Autodesk Inventor part; units mm, degrees
(part 3 of 3)
  spline S534 degree 2 poles (14.1065, -35.038) (14.0102, -34.9886) (13.7829, -34.959) (13.573, -34.959) knots 0 0 0 1 2 2 2
  line L552 (13.573, -34.959) -> (13.1135, -34.959)
  line L553 (13.1135, -34.959) -> (13.1135, -36.0853)
  line L554 (13.1135, -36.0853) -> (13.4421, -36.0853)
  spline S535 degree 2 poles (13.4421, -36.0853) (13.7088, -36.0853) (14.0151, -36.0359) (14.1337, -35.9568) knots 0 0 0 1 2 2 2
  spline S536 degree 2 poles (14.1337, -35.9568) (14.2473, -35.8753) (14.3535, -35.6728) (14.3535, -35.5122) knots 0 0 0 1 2 2 2
  spline S537 degree 2 poles (14.2102, -34.1266) (14.2102, -34.0179) (14.1361, -33.8549) (14.0546, -33.8079) knots 0 0 0 1 2 2 2
  spline S538 degree 2 poles (14.0546, -33.8079) (13.9558, -33.7536) (13.7162, -33.7289) (13.5013, -33.7289) knots 0 0 0 1 2 2 2
  line L555 (13.5013, -33.7289) -> (13.1135, -33.7289)
  line L556 (13.1135, -33.7289) -> (13.1135, -34.6206)
  line L557 (13.1135, -34.6206) -> (13.573, -34.6206)
  spline S539 degree 2 poles (13.573, -34.6206) (13.7632, -34.6206) (13.9435, -34.581) (14.0398, -34.5193) knots 0 0 0 1 2 2 2
  spline S540 degree 2 poles (14.0398, -34.5193) (14.1337, -34.46) (14.2102, -34.2698) (14.2102, -34.1266) knots 0 0 0 1 2 2 2
  spline S541 degree 2 poles (16.4234, -36.189) (16.3764, -36.2236) (16.2184, -36.3471) (16.1443, -36.3841) knots 0 0 0 1 2 2 2
  spline S542 degree 2 poles (16.1443, -36.3841) (16.043, -36.4385) (15.8528, -36.4953) (15.6799, -36.4953) knots 0 0 0 1 2 2 2
  spline S543 degree 2 poles (15.6799, -36.4953) (15.5391, -36.4953) (15.2847, -36.3891) (15.1884, -36.2928) knots 0 0 0 1 2 2 2
  spline S544 degree 2 poles (15.1884, -36.2928) (15.097, -36.1989) (14.9858, -35.9223) (14.9858, -35.7691) knots 0 0 0 1 2 2 2
  spline S545 degree 2 poles (14.9858, -35.7691) (14.9858, -35.532) (15.1859, -35.1961) (15.4032, -35.0997) knots 0 0 0 1 2 2 2
  spline S546 degree 2 poles (15.4032, -35.0997) (15.5959, -35.0108) (16.1195, -34.9441) (16.4234, -34.9268) knots 0 0 0 1 2 2 2
  line L558 (16.4234, -34.9268) -> (16.4234, -34.8527)
  spline S547 degree 2 poles (16.4234, -34.8527) (16.4234, -34.7194) (16.3419, -34.5539) (16.2678, -34.5069) knots 0 0 0 1 2 2 2
  spline S548 degree 2 poles (16.2678, -34.5069) (16.1937, -34.46) (15.9812, -34.4304) (15.8676, -34.4304) knots 0 0 0 1 2 2 2
  spline S549 degree 2 poles (15.8676, -34.4304) (15.7342, -34.4304) (15.3736, -34.5094) (15.1933, -34.586) knots 0 0 0 1 2 2 2
  line L559 (15.1933, -34.586) -> (15.1711, -34.586)
  line L560 (15.1711, -34.586) -> (15.1711, -34.1932)
  spline S550 degree 2 poles (15.1711, -34.1932) (15.2773, -34.1636) (15.6749, -34.0895) (15.8701, -34.0895) knots 0 0 0 1 2 2 2
  spline S551 degree 2 poles (15.8701, -34.0895) (16.1072, -34.0895) (16.4308, -34.1636) (16.5592, -34.2599) knots 0 0 0 1 2 2 2
  spline S552 degree 2 poles (16.5592, -34.2599) (16.6852, -34.3538) (16.8087, -34.6527) (16.8087, -34.8676) knots 0 0 0 1 2 2 2
  line L561 (16.8087, -34.8676) -> (16.8087, -36.4311)
  line L562 (16.8087, -36.4311) -> (16.4234, -36.4311)
  line L563 (16.4234, -36.4311) -> (16.4234, -36.189)
  line L564 (16.4234, -35.8679) -> (16.4234, -35.2331)
  spline S553 degree 2 poles (16.4234, -35.2331) (16.285, -35.2455) (15.8676, -35.2875) (15.7367, -35.327) knots 0 0 0 1 2 2 2
  spline S554 degree 2 poles (15.7367, -35.327) (15.5836, -35.3739) (15.3835, -35.569) (15.3835, -35.7419) knots 0 0 0 1 2 2 2
  spline S555 degree 2 poles (15.3835, -35.7419) (15.3835, -35.9395) (15.6058, -36.1396) (15.8182, -36.1396) knots 0 0 0 1 2 2 2
  spline S556 degree 2 poles (15.8182, -36.1396) (15.9985, -36.1396) (16.2949, -35.984) (16.4234, -35.8679) knots 0 0 0 1 2 2 2
  line L565 (18.5624, -34.5563) -> (18.5426, -34.5563)
  spline S557 degree 2 poles (18.5426, -34.5563) (18.4982, -34.544) (18.4018, -34.539) (18.3352, -34.539) knots 0 0 0 1 2 2 2
  spline S558 degree 2 poles (18.3352, -34.539) (18.1795, -34.539) (17.8733, -34.6749) (17.7349, -34.8083) knots 0 0 0 1 2 2 2
  line L566 (17.7349, -34.8083) -> (17.7349, -36.4311)
  line L567 (17.7349, -36.4311) -> (17.3496, -36.4311)
  line L568 (17.3496, -36.4311) -> (17.3496, -34.1438)
  line L569 (17.3496, -34.1438) -> (17.7349, -34.1438)
  line L570 (17.7349, -34.1438) -> (17.7349, -34.4847)
  spline S559 degree 2 poles (17.7349, -34.4847) (17.9449, -34.297) (18.2586, -34.1438) (18.4068, -34.1438) knots 0 0 0 1 2 2 2
  spline S560 degree 2 poles (18.4068, -34.1438) (18.4661, -34.1438) (18.5253, -34.1488) (18.5624, -34.1562) knots 0 0 0 1 2 2 2
  line L571 (18.5624, -34.1562) -> (18.5624, -34.5563)
  spline S561 degree 2 poles (19.7702, -36.483) (19.5331, -36.483) (19.1404, -36.3372) (18.9996, -36.189) knots 0 0 0 1 2 2 2
  spline S562 degree 2 poles (18.9996, -36.189) (18.8588, -36.0433) (18.7032, -35.5937) (18.7032, -35.2924) knots 0 0 0 1 2 2 2
  spline S563 degree 2 poles (18.7032, -35.2924) (18.7032, -34.9911) (18.8637, -34.5514) (18.9996, -34.4032) knots 0 0 0 1 2 2 2
  spline S564 degree 2 poles (18.9996, -34.4032) (19.1354, -34.2525) (19.5381, -34.092) (19.7702, -34.092) knots 0 0 0 1 2 2 2
  spline S565 degree 2 poles (19.7702, -34.092) (19.958, -34.092) (20.3087, -34.1982) (20.4445, -34.2673) knots 0 0 0 1 2 2 2
  line L572 (20.4445, -34.2673) -> (20.4445, -34.6996)
  line L573 (20.4445, -34.6996) -> (20.4223, -34.6996)
  spline S566 degree 2 poles (20.4223, -34.6996) (20.3803, -34.665) (20.2519, -34.5761) (20.1605, -34.5292) knots 0 0 0 1 2 2 2
  spline S567 degree 2 poles (20.1605, -34.5292) (20.079, -34.4896) (19.8616, -34.4279) (19.7628, -34.4279) knots 0 0 0 1 2 2 2
  spline S568 degree 2 poles (19.7628, -34.4279) (19.464, -34.4279) (19.1009, -34.8799) (19.1009, -35.2924) knots 0 0 0 1 2 2 2
  spline S569 degree 2 poles (19.1009, -35.2924) (19.1009, -35.695) (19.4516, -36.147) (19.7628, -36.147) knots 0 0 0 1 2 2 2
  spline S570 degree 2 poles (19.7628, -36.147) (19.9505, -36.147) (20.2914, -35.9914) (20.4223, -35.8704) knots 0 0 0 1 2 2 2
  line L574 (20.4223, -35.8704) -> (20.4445, -35.8704)
  line L575 (20.4445, -35.8704) -> (20.4445, -36.3026)
  spline S571 degree 2 poles (20.4445, -36.3026) (20.3877, -36.3298) (20.2148, -36.4064) (20.1457, -36.4237) knots 0 0 0 1 2 2 2
  spline S572 degree 2 poles (20.1457, -36.4237) (20.0469, -36.4533) (19.8913, -36.483) (19.7702, -36.483) knots 0 0 0 1 2 2 2
  spline S573 degree 2 poles (21.7882, -36.483) (21.2399, -36.483) (20.6372, -35.8679) (20.6372, -35.2998) knots 0 0 0 1 2 2 2
  spline S574 degree 2 poles (20.6372, -35.2998) (20.6372, -34.7416) (21.2226, -34.0796) (21.6944, -34.0796) knots 0 0 0 1 2 2 2
  spline S575 degree 2 poles (21.6944, -34.0796) (21.9068, -34.0796) (22.2353, -34.2031) (22.3563, -34.334) knots 0 0 0 1 2 2 2
  spline S576 degree 2 poles (22.3563, -34.334) (22.4798, -34.4649) (22.6108, -34.8429) (22.6108, -35.117) knots 0 0 0 1 2 2 2
  line L576 (22.6108, -35.117) -> (22.6108, -35.327)
  line L577 (22.6108, -35.327) -> (21.0275, -35.327)
  spline S577 degree 2 poles (21.0275, -35.327) (21.0275, -35.7247) (21.4276, -36.147) (21.7833, -36.147) knots 0 0 0 1 2 2 2
  spline S578 degree 2 poles (21.7833, -36.147) (21.9093, -36.147) (22.1538, -36.0902) (22.2526, -36.0458) knots 0 0 0 1 2 2 2
  spline S579 degree 2 poles (22.2526, -36.0458) (22.3563, -35.9964) (22.4996, -35.9099) (22.5465, -35.8704) knots 0 0 0 1 2 2 2
  line L578 (22.5465, -35.8704) -> (22.5688, -35.8704)
  line L579 (22.5688, -35.8704) -> (22.5688, -36.2903)
  spline S580 degree 2 poles (22.5688, -36.2903) (22.5021, -36.3175) (22.2995, -36.3965) (22.2205, -36.4187) knots 0 0 0 1 2 2 2
  spline S581 degree 2 poles (22.2205, -36.4187) (22.1093, -36.4508) (21.9266, -36.483) (21.7882, -36.483) knots 0 0 0 1 2 2 2
  spline S582 degree 2 poles (22.2353, -35.0331) (22.2304, -34.8774) (22.1661, -34.6502) (22.1044, -34.5736) knots 0 0 0 1 2 2 2
  spline S583 degree 2 poles (22.1044, -34.5736) (22.0377, -34.4872) (21.8278, -34.3958) (21.6721, -34.3958) knots 0 0 0 1 2 2 2
  spline S584 degree 2 poles (21.6721, -34.3958) (21.519, -34.3958) (21.3041, -34.4872) (21.2152, -34.5761) knots 0 0 0 1 2 2 2
  spline S585 degree 2 poles (21.2152, -34.5761) (21.1287, -34.6675) (21.0398, -34.8873) (21.0275, -35.0331) knots 0 0 0 1 2 2 2
  line L580 (21.0275, -35.0331) -> (22.2353, -35.0331)
  line L581 (23.3937, -36.4311) -> (23.0084, -36.4311)
  line L582 (23.0084, -36.4311) -> (23.0084, -33.2472)
  line L583 (23.0084, -33.2472) -> (23.3937, -33.2472)
  line L584 (23.3937, -33.2472) -> (23.3937, -36.4311)
  line L585 (24.3521, -36.4311) -> (23.9668, -36.4311)
  line L586 (23.9668, -36.4311) -> (23.9668, -33.2472)
  line L587 (23.9668, -33.2472) -> (24.3521, -33.2472)
  line L588 (24.3521, -33.2472) -> (24.3521, -36.4311)
  spline S586 degree 2 poles (26.7974, -35.2875) (26.7974, -35.8654) (26.2417, -36.4953) (25.7773, -36.4953) knots 0 0 0 1 2 2 2
  spline S587 degree 2 poles (25.7773, -36.4953) (25.3006, -36.4953) (24.7547, -35.8457) (24.7547, -35.2875) knots 0 0 0 1 2 2 2
  spline S588 degree 2 poles (24.7547, -35.2875) (24.7547, -34.7144) (25.3179, -34.0796) (25.7773, -34.0796) knots 0 0 0 1 2 2 2
  spline S589 degree 2 poles (25.7773, -34.0796) (26.2417, -34.0796) (26.7974, -34.7119) (26.7974, -35.2875) knots 0 0 0 1 2 2 2
  spline S590 degree 2 poles (26.3998, -35.2875) (26.3998, -34.8429) (26.0762, -34.4106) (25.7773, -34.4106) knots 0 0 0 1 2 2 2
  spline S591 degree 2 poles (25.7773, -34.4106) (25.4784, -34.4106) (25.1524, -34.8429) (25.1524, -35.2875) knots 0 0 0 1 2 2 2
  spline S592 degree 2 poles (25.1524, -35.2875) (25.1524, -35.7197) (25.4784, -36.1643) (25.7773, -36.1643) knots 0 0 0 1 2 2 2
  spline S593 degree 2 poles (25.7773, -36.1643) (26.0737, -36.1643) (26.3998, -35.7271) (26.3998, -35.2875) knots 0 0 0 1 2 2 2
  point P0 (0, 0)
  constraints: 4 other
extrude "Extrusion6" cut sketch "Sketch2" against normal blind 0.25
body "Solid1"
